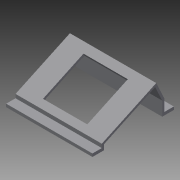
# Autodesk Inventor part: DisplayMount
Saved by Autodesk Inventor 2015 (Build 190159000, 159)
## iProperties
Created: 2022-04-16
Part Number: DisplayMount
Material: Generic
Document SubType Name: Modeling
Designer: Jan
Density: 1 g/cm^3
Appearance: Default
Author: Jan
Autodesk Inventor part; units mm, degrees
ref_plane "YZ Plane" through (0, 0, 0) normal (1, 0, 0) x (0, 1, 0)
ref_plane "XZ Plane" through (0, 0, 0) normal (0, 1, 0) x (-1, 0, 0)
ref_plane "XY Plane" through (0, 0, 0) normal (0, 0, 1) x (1, 0, 0)
sketch "Sketch1" plane through (0, 0, 0) normal (1, 0, 0) x (0, 1, 0)
  line L0 (-1.2, 3.6) -> (27.8018, 17.1238)
  line L1 (27.8018, 17.1238) -> (32.2, 7.6919)
  line L2 (37.2, 1.6) -> (37.2, 0)
  line L3 (37.2, 0) -> (31, 0)
  line L4 (31, 0) -> (31, 7.4259)
  line L5 (31, 7.4259) -> (27.2214, 15.5291)
  line L6 (27.2214, 15.5291) -> (0, 2.8355)
  line L7 (0, 2.8355) -> (0, 0)
  line L8 (-6.2, 0) -> (-6.2, 1.6)
  line L9 (-1.2, 3.6) -> (-1.2, 1.6)
  line L10 (-1.2, 1.6) -> (-6.2, 1.6)
  line L11 (32.2, 7.6919) -> (32.2, 1.6)
  line L12 (32.2, 1.6) -> (37.2, 1.6)
  line L13 (-6.2, 0) -> (0, 0)
  dimension "d0" = 1.2
  dimension "d1" = 1.2
  dimension "d2" = 31
  dimension "d3" = 1.2
  dimension "d4" = 1.2
  dimension "d5" = 2
  dimension "d6" = 25
  dimension "d7" = 1.6
  dimension "d9" = 5
  dimension "d25" = 32
  constraints: 28 end point, 4 vertical, 3 collinear, 3 horizontal, 3 parallel, 2 perpendicular, 1 coincident
  measures "d0" distance between parallel lines of L9 L7
  measures "d1" distance between parallel lines of L4 L11
  measures "d2" distance between parallel lines of L4 L7
  measures "d3" distance between parallel lines of L6 L0
  measures "d4" distance between parallel lines of L1 L5
  measures "d5" distance of L0.start L9.end
  measures "d6" angle of L6 L13
  measures "d7" distance between parallel lines of L13 L10
  measures "d9" distance of L9.end L8.end
  measures "d25" distance of L0.start L0.end
extrude "Extrusion1" add sketch "Sketch1" along normal blind 46
sketch "Sketch3" plane through (46, 27.2214, 15.5291) normal (0, 0.4226183, -0.9063078) x (-1, 0, 0)
  circle A0 centre (3.405, -3.2297) radius 1.05
  circle A1 centre (37.695, -3.2297) radius 1.05
  circle A2 centre (37.695, -26.1407) radius 1.05
  circle A3 centre (3.405, -26.1407) radius 1.05
  line L0 (0, -30.0355) -> (0, 0) construction
  line L1 (46, -30.0355) -> (46, 0) construction
  circle A4 centre (3.405, -3.2297) radius 1.85
  circle A5 centre (37.695, -3.2297) radius 1.85
  circle A6 centre (37.695, -26.1407) radius 1.85
  circle A7 centre (3.405, -26.1407) radius 1.85
  line L2 (11.205, -3.1832) -> (34.795, -3.1832)
  line L3 (34.795, -3.1832) -> (34.795, -26.9832)
  line L4 (34.795, -26.9832) -> (11.205, -26.9832)
  line L5 (11.205, -26.9832) -> (11.205, -3.1832)
  line L6 (23, -3.1832) -> (23, -26.9832) construction
  line L7 (11.205, -15.0832) -> (0, -15.0832) construction
  line L8 (34.795, -15.0832) -> (46, -15.0832) construction
  point P0 (46, -31.2339)
  dimension "d13" = 34.29
  dimension "d14" = 22.911
  dimension "d15" = 2.1
  dimension "d16" = 0.8
  dimension "d17" = 7.8
  dimension "d18" = 2.9
  dimension "d19" = 23.8
  constraints: 14 end point, 8 centre point, 6 equal radius, 4 coincident, 4 midpoint, 3 perpendicular, 2 horizontal alignment, 2 parallel, 2 point on line, 2 vertical alignment, 1 collinear, 1 horizontal
  measures "d13" distance of A1.centre A0.centre
  measures "d14" distance of A3.centre A0.centre
  measures "d15" diameter of A0
  measures "d16" radial gap between concentric circles of A4 A0
  measures "d17" distance from line of L5 A0.centre
  measures "d18" distance from line of A1.centre L3
  measures "d19" distance between parallel lines of L4 L2
extrude "Extrusion2" add sketch "Sketch3" along normal blind 1.7 contours A4 | A5 | A6 | A7
extrude "Extrusion3" cut sketch "Sketch3" against normal up to surface (1.2 mm away) contours L2 L3 L4 L5
body "Solid1"
